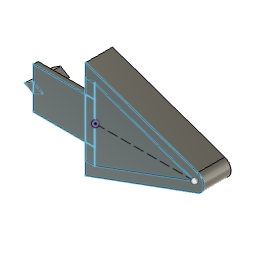
diagonal_cutter_cover (Autodesk Fusion 360 design; units mm, degrees)
Autodesk Fusion 360 part; units mm, degrees
sketch "Sketch1" plane through (0, 0, 0) normal (0, 1, 0) x (1, 0, 0)
  line L0 (-0.1521, 9.4703) -> (-0.1521, -9.0297)
  line L1 (0, 0) -> (25.7, 0) construction
  line L2 (-0.1521, -9.0297) -> (25.7, 0)
  line L3 (-0.1521, 9.4703) -> (25.7, 0)
  line L4 (-2.5521, 12.9054) -> (26.5255, 2.2536)
  line L5 (-2.5521, -12.4102) -> (26.4914, -2.2658)
  line L6 (-2.5521, 12.9054) -> (-2.5521, -12.4102)
  arc A0 (26.4914, -2.2658) -> (26.5255, 2.2536) centre (25.7, 0) ccw
  line L7 (-0.1521, -9.0297) -> (-2.5521, -9.0297)
  line L8 (-2.5521, -9.0297) -> (-2.5521, 9.4703)
  line L9 (-2.5521, 9.4703) -> (-0.1521, 9.4703)
  line L10 (-0.1521, 9.4703) -> (-0.1521, -9.0297)
  line L11 (-0.1521, -5.334) -> (-16.0521, -5.334)
  line L12 (-16.0521, -5.334) -> (-16.0521, 5.366)
  line L13 (-16.0521, 5.366) -> (-0.1521, 5.366)
  line L14 (-0.1521, 5.366) -> (-0.1521, -5.334)
  line L15 (-18.2359, 0.016) -> (-13.6958, 0.016) construction
  line L16 (-16.0521, -1.3788) -> (-16.0521, 1.1212) construction
  line L17 (-16.0521, -1.3788) -> (-18.2359, 0.016)
  line L18 (-18.2359, 0.016) -> (-16.0521, 1.1212)
  line L19 (-16.0521, 1.1212) -> (-13.6958, 0.016)
  line L20 (-13.6958, 0.016) -> (-16.0521, -1.3788)
  dimension "d1" = 18.5
  dimension "d2" = 25.7
  dimension "d4" = 2.4
  dimension "d5" = 2.4
  dimension "d6" = 18.5
  dimension "d7" = 15.9
  dimension "d8" = 10.7
  dimension "d9" = 2.5
  constraint vertical L0
  constraint coincident L1.start origin
  constraint perpendicular L0 L1
  constraint parallel L3 L4
  constraint parallel L2 L5
  constraint parallel L0 L6
  constraint tangent L4 A0
  constraint tangent L5 A0
  constraint horizontal L7
  constraint vertical L8
  constraint horizontal L9
  constraint vertical L10
  constraint horizontal L11
  constraint vertical L12
  constraint horizontal L13
  constraint vertical L14
  constraint coincident L0 L11.start
  constraint perpendicular L12 L15
  constraint coincident L12 L16.start
  constraint perpendicular L15 L16
  measures "d1" distance of L0.start L0.end
  measures "d2" distance of L1.start L1.end
  measures "d4" radius of A0
  measures "d5" distance of L0.end L7.end
  measures "d6" distance of L0.end L0.start
  measures "d7" distance of L11.start L11.end
  measures "d8" distance of L11.start L13.end
  measures "d9" distance of L16.start L16.end
extrude "Extrude2" add sketch "Sketch1" along normal blind 1.2 contours L0 L2 L3 L10 L14 | L0 L6 L8 L9 L10 L13 | L0 L6 L8 L10 L11 L13 L14 | L0 L6 L7 L8 L10 L11 | L6 L8 L11 L12 L13 L19 L20 makes body 1
extrude "Extrude1" add sketch "Sketch1" along normal blind 7 separate body contours L2 L3 L4 L5 L6 A0 L7 L9 | L12 L19 L20 | L12 L17 L18 makes body 2 at (-14.4813, 2.3333, 0.449) makes body 3 at (7.1404, 2.3333, -9.3548)
